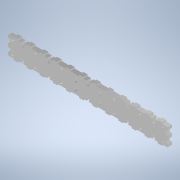
# Autodesk Inventor part: BackWallFrame
Saved by Autodesk Inventor 2021 (Build 250183000, 183)
## iProperties
Created: 2021-03-05
Part Number: BackWallFrame
Material: Aluminum 6061
Document SubType Name: Modeling
Designer: M3rob
Mass: 6286.27 g
Surface Area: 2801.63 cm^2
Volume: 2328.25 cm^3
Density: 2.7 g/cm^3
Appearance: Aluminum - Flat
Author: M3rob
Autodesk Inventor part; units mm, degrees
ref_plane "YZ Plane" through (0, 0, 0) normal (1, 0, 0) x (0, 1, 0)
ref_plane "XZ Plane" through (0, 0, 0) normal (0, 1, 0) x (-1, 0, 0)
ref_plane "XY Plane" through (0, 0, 0) normal (0, 0, 1) x (1, 0, 0)
sketch "Sketch1" plane through (0, 0, 0) normal (0, 0, 1) x (1, 0, 0)
  line L0 (-463.55, 50.8) -> (-431.8, 50.8)
  line L1 (463.55, 50.8) -> (463.55, 34.8615)
  line L2 (463.55, -50.8) -> (-463.55, -50.8)
  line L3 (-463.55, -50.8) -> (-463.55, -34.8615)
  line L4 (-463.55, 34.8615) -> (-450.85, 34.8615)
  line L5 (-450.85, 34.8615) -> (-450.85, 9.4615)
  line L6 (-450.85, 9.4615) -> (-463.55, 9.4615)
  line L7 (-463.55, -9.4615) -> (-450.85, -9.4615)
  line L8 (-450.85, -9.4615) -> (-450.85, -34.8615)
  line L9 (-450.85, -34.8615) -> (-463.55, -34.8615)
  line L10 (-463.55, 0) -> (0, 0) construction
  line L11 (0, 0) -> (0, 50.8) construction
  line L12 (-463.55, 34.8615) -> (-463.55, 50.8)
  line L13 (-463.55, 9.4615) -> (-463.55, 34.8615) construction
  line L14 (-463.55, -9.4615) -> (-463.55, 9.4615)
  line L15 (-463.55, -34.8615) -> (-463.55, -9.4615) construction
  line L16 (463.55, 34.8615) -> (450.85, 34.8615)
  line L17 (450.85, 34.8615) -> (450.85, 9.4615)
  line L18 (450.85, 9.4615) -> (463.55, 9.4615)
  line L19 (463.55, -9.4615) -> (450.85, -9.4615)
  line L20 (450.85, -9.4615) -> (450.85, -34.8615)
  line L21 (450.85, -34.8615) -> (463.55, -34.8615)
  line L22 (463.55, 9.4615) -> (463.55, -9.4615)
  line L23 (463.55, 34.8615) -> (463.55, 9.4615) construction
  line L24 (463.55, -9.4615) -> (463.55, -34.8615) construction
  line L25 (463.55, -34.8615) -> (463.55, -50.8)
  line L26 (-76.2, 34.8615) -> (-63.5, 34.8615)
  line L27 (-63.5, 34.8615) -> (-63.5, 9.4615)
  line L28 (-63.5, 9.4615) -> (-76.2, 9.4615)
  line L29 (-76.2, 9.4615) -> (-76.2, 34.8615)
  line L30 (-76.2, -9.4615) -> (-63.5, -9.4615)
  line L31 (-63.5, -9.4615) -> (-63.5, -34.8615)
  line L32 (-63.5, -34.8615) -> (-76.2, -34.8615)
  line L33 (-76.2, -34.8615) -> (-76.2, -9.4615)
  line L34 (76.2, -9.4615) -> (63.5, -9.4615)
  line L35 (63.5, -9.4615) -> (63.5, -34.8615)
  line L36 (63.5, -34.8615) -> (76.2, -34.8615)
  line L37 (76.2, -34.8615) -> (76.2, -9.4615)
  line L38 (76.2, 34.8615) -> (63.5, 34.8615)
  line L39 (63.5, 34.8615) -> (63.5, 9.4615)
  line L40 (63.5, 9.4615) -> (76.2, 9.4615)
  line L41 (76.2, 9.4615) -> (76.2, 34.8615)
  line L42 (-431.8, 50.8) -> (-431.8, 58.7375)
  line L43 (-431.8, 58.7375) -> (-406.4, 58.7375)
  line L44 (-406.4, 58.7375) -> (-406.4, 50.8)
  line L45 (-355.6, 50.8) -> (-355.6, 58.7375)
  line L46 (-355.6, 58.7375) -> (-330.2, 58.7375)
  line L47 (-330.2, 58.7375) -> (-330.2, 50.8)
  line L48 (-279.4, 50.8) -> (-279.4, 58.7375)
  line L49 (-279.4, 58.7375) -> (-254, 58.7375)
  line L50 (-254, 58.7375) -> (-254, 50.8)
  line L51 (-203.2, 50.8) -> (-203.2, 58.7375)
  line L52 (-203.2, 58.7375) -> (-177.8, 58.7375)
  line L53 (-177.8, 58.7375) -> (-177.8, 50.8)
  line L54 (-431.8, 50.8) -> (-406.4, 50.8) construction
  line L55 (-406.4, 50.8) -> (-387.7437, 50.8)
  line L56 (-355.6, 50.8) -> (-330.2, 50.8) construction
  line L57 (-330.2, 50.8) -> (-279.4, 50.8)
  line L58 (-254, 50.8) -> (-203.2, 50.8)
  line L59 (-279.4, 50.8) -> (-254, 50.8) construction
  line L60 (-177.8, 50.8) -> (463.55, 50.8)
  line L61 (-203.2, 50.8) -> (-177.8, 50.8) construction
  line L62 (-127, 58.7375) -> (-101.6, 58.7375)
  line L63 (-101.6, 58.7375) -> (-101.6, 50.8)
  line L64 (-101.6, 50.8) -> (-127, 50.8)
  line L65 (-127, 50.8) -> (-127, 50.8)
  line L66 (-127, 50.8) -> (-127, 58.7375)
  line L67 (-50.8, 50.8) -> (-50.8, 58.7375)
  line L68 (-50.8, 50.8) -> (-50.8, 50.8)
  line L69 (-25.4, 50.8) -> (-50.8, 50.8)
  line L70 (-25.4, 58.7375) -> (-25.4, 50.8)
  line L71 (-50.8, 58.7375) -> (-25.4, 58.7375)
  line L72 (25.4, 50.8) -> (25.4, 58.7375)
  line L73 (25.4, 50.8) -> (25.4, 50.8)
  line L74 (50.8, 50.8) -> (25.4, 50.8)
  line L75 (50.8, 58.7375) -> (50.8, 50.8)
  line L76 (25.4, 58.7375) -> (50.8, 58.7375)
  line L77 (101.6, 50.8) -> (101.6, 58.7375)
  line L78 (101.6, 50.8) -> (101.6, 50.8)
  line L79 (127, 50.8) -> (101.6, 50.8)
  line L80 (127, 58.7375) -> (127, 50.8)
  line L81 (101.6, 58.7375) -> (127, 58.7375)
  line L82 (177.8, 50.8) -> (177.8, 58.7375)
  line L83 (177.8, 50.8) -> (177.8, 50.8)
  line L84 (203.2, 50.8) -> (177.8, 50.8)
  line L85 (203.2, 58.7375) -> (203.2, 50.8)
  line L86 (177.8, 58.7375) -> (203.2, 58.7375)
  line L87 (254, 50.8) -> (254, 58.7375)
  line L88 (254, 50.8) -> (254, 50.8)
  line L89 (279.4, 50.8) -> (254, 50.8)
  line L90 (279.4, 58.7375) -> (279.4, 50.8)
  line L91 (254, 58.7375) -> (279.4, 58.7375)
  line L92 (330.2, 50.8) -> (330.2, 58.7375)
  line L93 (330.2, 50.8) -> (330.2, 50.8)
  line L94 (355.6, 50.8) -> (330.2, 50.8)
  line L95 (355.6, 58.7375) -> (355.6, 50.8)
  line L96 (330.2, 58.7375) -> (355.6, 58.7375)
  line L97 (406.4, 50.8) -> (406.4, 58.7375)
  line L98 (406.4, 50.8) -> (406.4, 50.8)
  line L99 (431.8, 50.8) -> (406.4, 50.8)
  line L100 (431.8, 58.7375) -> (431.8, 50.8)
  line L101 (406.4, 58.7375) -> (431.8, 58.7375)
  line L102 (431.8, 58.7375) -> (463.55, 50.8) construction
  line L103 (-431.8, 58.7375) -> (-463.55, 50.8) construction
  line L104 (-431.8, -50.8) -> (-431.8, -58.7375)
  line L105 (-431.8, -58.7375) -> (-406.4, -58.7375)
  line L106 (-406.4, -58.7375) -> (-406.4, -50.8)
  line L107 (-355.6, -50.8) -> (-355.6, -58.7375)
  line L108 (-355.6, -58.7375) -> (-330.2, -58.7375)
  line L109 (-330.2, -58.7375) -> (-330.2, -50.8)
  line L110 (-279.4, -50.8) -> (-279.4, -58.7375)
  line L111 (-279.4, -58.7375) -> (-254, -58.7375)
  line L112 (-254, -58.7375) -> (-254, -50.8)
  line L113 (-203.2, -50.8) -> (-203.2, -58.7375)
  line L114 (-203.2, -58.7375) -> (-177.8, -58.7375)
  line L115 (-177.8, -58.7375) -> (-177.8, -50.8)
  line L116 (-431.8, -50.8) -> (-406.4, -50.8) construction
  line L117 (-355.6, -50.8) -> (-330.2, -50.8) construction
  line L118 (-279.4, -50.8) -> (-254, -50.8) construction
  line L119 (-203.2, -50.8) -> (-177.8, -50.8) construction
  line L120 (-127, -58.7375) -> (-101.6, -58.7375)
  line L121 (-101.6, -58.7375) -> (-101.6, -50.8)
  line L122 (-101.6, -50.8) -> (-127, -50.8)
  line L123 (-127, -50.8) -> (-127, -58.7375)
  line L124 (-50.8, -50.8) -> (-50.8, -58.7375)
  line L125 (-25.4, -50.8) -> (-50.8, -50.8)
  line L126 (-25.4, -58.7375) -> (-25.4, -50.8)
  line L127 (-50.8, -58.7375) -> (-25.4, -58.7375)
  line L128 (25.4, -50.8) -> (25.4, -58.7375)
  line L129 (50.8, -50.8) -> (25.4, -50.8)
  line L130 (50.8, -58.7375) -> (50.8, -50.8)
  line L131 (25.4, -58.7375) -> (50.8, -58.7375)
  line L132 (101.6, -50.8) -> (101.6, -58.7375)
  line L133 (127, -50.8) -> (101.6, -50.8)
  line L134 (127, -58.7375) -> (127, -50.8)
  line L135 (101.6, -58.7375) -> (127, -58.7375)
  line L136 (177.8, -50.8) -> (177.8, -58.7375)
  line L137 (203.2, -50.8) -> (177.8, -50.8)
  line L138 (203.2, -58.7375) -> (203.2, -50.8)
  line L139 (177.8, -58.7375) -> (203.2, -58.7375)
  line L140 (254, -50.8) -> (254, -58.7375)
  line L141 (279.4, -50.8) -> (254, -50.8)
  line L142 (279.4, -58.7375) -> (279.4, -50.8)
  line L143 (254, -58.7375) -> (279.4, -58.7375)
  line L144 (330.2, -50.8) -> (330.2, -58.7375)
  line L145 (355.6, -50.8) -> (330.2, -50.8)
  line L146 (355.6, -58.7375) -> (355.6, -50.8)
  line L147 (330.2, -58.7375) -> (355.6, -58.7375)
  line L148 (406.4, -50.8) -> (406.4, -58.7375)
  line L149 (431.8, -50.8) -> (406.4, -50.8)
  line L150 (431.8, -58.7375) -> (431.8, -50.8)
  line L151 (406.4, -58.7375) -> (431.8, -58.7375)
  line L152 (-387.7437, 50.8) -> (-387.7437, 41.275)
  line L153 (-387.7437, 41.275) -> (-390.525, 41.275)
  line L154 (-390.525, 41.275) -> (-390.525, 30.1625)
  line L155 (-390.525, 30.1625) -> (-387.7437, 30.1625)
  line L156 (-387.7437, 30.1625) -> (-387.7437, 26.9875)
  line L157 (-387.7437, 26.9875) -> (-374.2563, 26.9875)
  line L158 (-374.2563, 26.9875) -> (-374.2563, 30.1625)
  line L159 (-374.2563, 30.1625) -> (-371.475, 30.1625)
  line L160 (-371.475, 30.1625) -> (-371.475, 41.275)
  line L161 (-371.475, 41.275) -> (-374.2563, 41.275)
  line L162 (-381, 50.8) -> (-381, 26.9875) construction
  line L163 (-374.2563, 41.275) -> (-374.2563, 50.8)
  line L164 (-387.7437, 50.8) -> (-374.2563, 50.8)
  line L165 (-374.2563, 50.8) -> (-355.6, 50.8)
  line L166 (-387.7437, -50.8) -> (-387.7437, -41.275)
  line L167 (-387.7437, -41.275) -> (-390.525, -41.275)
  line L168 (-390.525, -41.275) -> (-390.525, -30.1625)
  line L169 (-390.525, -30.1625) -> (-387.7437, -30.1625)
  line L170 (-387.7437, -30.1625) -> (-387.7437, -26.9875)
  line L171 (-387.7437, -26.9875) -> (-374.2563, -26.9875)
  line L172 (-374.2563, -26.9875) -> (-374.2563, -30.1625)
  line L173 (-374.2563, -30.1625) -> (-371.475, -30.1625)
  line L174 (-371.475, -30.1625) -> (-371.475, -41.275)
  line L175 (-371.475, -41.275) -> (-374.2563, -41.275)
  line L176 (-381, -50.8) -> (-381, -26.9875) construction
  line L177 (-374.2563, -41.275) -> (-374.2563, -50.8)
  line L178 (-387.7437, -50.8) -> (-374.2563, -50.8)
  line L179 (-314.325, 41.275) -> (-314.325, 30.1625)
  line L180 (-314.325, 30.1625) -> (-311.5437, 30.1625)
  line L181 (-311.5437, 30.1625) -> (-311.5437, 26.9875)
  line L182 (-304.8, 50.8) -> (-304.8, 26.9875) construction
  line L183 (-311.5437, 50.8) -> (-298.0563, 50.8)
  line L184 (-298.0563, 41.275) -> (-298.0563, 50.8)
  line L185 (-311.5437, 26.9875) -> (-298.0563, 26.9875)
  line L186 (-298.0563, 26.9875) -> (-298.0563, 30.1625)
  line L187 (-298.0563, 30.1625) -> (-295.275, 30.1625)
  line L188 (-295.275, 30.1625) -> (-295.275, 41.275)
  line L189 (-295.275, 41.275) -> (-298.0563, 41.275)
  line L190 (-311.5437, 50.8) -> (-311.5437, 41.275)
  line L191 (-311.5437, 41.275) -> (-314.325, 41.275)
  line L192 (-311.5437, -41.275) -> (-314.325, -41.275)
  line L193 (-311.5437, -50.8) -> (-311.5437, -41.275)
  line L194 (-314.325, -41.275) -> (-314.325, -30.1625)
  line L195 (-314.325, -30.1625) -> (-311.5437, -30.1625)
  line L196 (-311.5437, -30.1625) -> (-311.5437, -26.9875)
  line L197 (-311.5437, -50.8) -> (-298.0563, -50.8)
  line L198 (-304.8, -50.8) -> (-304.8, -26.9875) construction
  line L199 (-298.0563, -41.275) -> (-298.0563, -50.8)
  line L200 (-295.275, -41.275) -> (-298.0563, -41.275)
  line L201 (-311.5437, -26.9875) -> (-298.0563, -26.9875)
  line L202 (-295.275, -30.1625) -> (-295.275, -41.275)
  line L203 (-298.0563, -30.1625) -> (-295.275, -30.1625)
  line L204 (-298.0563, -26.9875) -> (-298.0563, -30.1625)
  line L205 (-238.125, 41.275) -> (-238.125, 30.1625)
  line L206 (-238.125, 30.1625) -> (-235.3437, 30.1625)
  line L207 (-235.3437, 30.1625) -> (-235.3437, 26.9875)
  line L208 (-228.6, 50.8) -> (-228.6, 26.9875) construction
  line L209 (-235.3437, 50.8) -> (-221.8563, 50.8)
  line L210 (-221.8563, 41.275) -> (-221.8563, 50.8)
  line L211 (-235.3437, 26.9875) -> (-221.8563, 26.9875)
  line L212 (-221.8563, 26.9875) -> (-221.8563, 30.1625)
  line L213 (-221.8563, 30.1625) -> (-219.075, 30.1625)
  line L214 (-219.075, 30.1625) -> (-219.075, 41.275)
  line L215 (-219.075, 41.275) -> (-221.8563, 41.275)
  line L216 (-235.3437, 50.8) -> (-235.3437, 41.275)
  line L217 (-235.3437, 41.275) -> (-238.125, 41.275)
  line L218 (-235.3437, -41.275) -> (-238.125, -41.275)
  line L219 (-235.3437, -50.8) -> (-235.3437, -41.275)
  line L220 (-238.125, -41.275) -> (-238.125, -30.1625)
  line L221 (-238.125, -30.1625) -> (-235.3437, -30.1625)
  line L222 (-235.3437, -30.1625) -> (-235.3437, -26.9875)
  line L223 (-235.3437, -50.8) -> (-221.8563, -50.8)
  line L224 (-228.6, -50.8) -> (-228.6, -26.9875) construction
  line L225 (-221.8563, -41.275) -> (-221.8563, -50.8)
  line L226 (-219.075, -41.275) -> (-221.8563, -41.275)
  line L227 (-235.3437, -26.9875) -> (-221.8563, -26.9875)
  line L228 (-219.075, -30.1625) -> (-219.075, -41.275)
  line L229 (-221.8563, -30.1625) -> (-219.075, -30.1625)
  line L230 (-221.8563, -26.9875) -> (-221.8563, -30.1625)
  line L231 (-161.925, 41.275) -> (-161.925, 30.1625)
  line L232 (-161.925, 30.1625) -> (-159.1437, 30.1625)
  line L233 (-159.1437, 30.1625) -> (-159.1437, 26.9875)
  line L234 (-152.4, 50.8) -> (-152.4, 26.9875) construction
  line L235 (-159.1437, 50.8) -> (-145.6563, 50.8)
  line L236 (-145.6563, 41.275) -> (-145.6563, 50.8)
  line L237 (-159.1437, 26.9875) -> (-145.6563, 26.9875)
  line L238 (-145.6563, 26.9875) -> (-145.6563, 30.1625)
  line L239 (-145.6563, 30.1625) -> (-142.875, 30.1625)
  line L240 (-142.875, 30.1625) -> (-142.875, 41.275)
  line L241 (-142.875, 41.275) -> (-145.6563, 41.275)
  line L242 (-159.1437, 50.8) -> (-159.1437, 41.275)
  line L243 (-159.1437, 41.275) -> (-161.925, 41.275)
  line L244 (-159.1437, -41.275) -> (-161.925, -41.275)
  line L245 (-159.1437, -50.8) -> (-159.1437, -41.275)
  line L246 (-161.925, -41.275) -> (-161.925, -30.1625)
  line L247 (-161.925, -30.1625) -> (-159.1437, -30.1625)
  line L248 (-159.1437, -30.1625) -> (-159.1437, -26.9875)
  line L249 (-159.1437, -50.8) -> (-145.6563, -50.8)
  line L250 (-152.4, -50.8) -> (-152.4, -26.9875) construction
  line L251 (-145.6563, -41.275) -> (-145.6563, -50.8)
  line L252 (-142.875, -41.275) -> (-145.6563, -41.275)
  line L253 (-159.1437, -26.9875) -> (-145.6563, -26.9875)
  line L254 (-142.875, -30.1625) -> (-142.875, -41.275)
  line L255 (-145.6563, -30.1625) -> (-142.875, -30.1625)
  line L256 (-145.6563, -26.9875) -> (-145.6563, -30.1625)
  line L257 (-85.725, 41.275) -> (-85.725, 30.1625)
  line L258 (-85.725, 30.1625) -> (-82.9437, 30.1625)
  line L259 (-82.9437, 30.1625) -> (-82.9437, 26.9875)
  line L260 (-76.2, 50.8) -> (-76.2, 26.9875) construction
  line L261 (-82.9437, 50.8) -> (-69.4563, 50.8)
  line L262 (-69.4563, 41.275) -> (-69.4563, 50.8)
  line L263 (-82.9437, 26.9875) -> (-69.4563, 26.9875)
  line L264 (-69.4563, 26.9875) -> (-69.4563, 30.1625)
  line L265 (-69.4563, 30.1625) -> (-66.675, 30.1625)
  line L266 (-66.675, 30.1625) -> (-66.675, 41.275)
  line L267 (-66.675, 41.275) -> (-69.4563, 41.275)
  line L268 (-82.9437, 50.8) -> (-82.9437, 41.275)
  line L269 (-82.9437, 41.275) -> (-85.725, 41.275)
  line L270 (-82.9437, -41.275) -> (-85.725, -41.275)
  line L271 (-82.9437, -50.8) -> (-82.9437, -41.275)
  line L272 (-85.725, -41.275) -> (-85.725, -30.1625)
  line L273 (-85.725, -30.1625) -> (-82.9437, -30.1625)
  line L274 (-82.9437, -30.1625) -> (-82.9437, -26.9875)
  line L275 (-82.9437, -50.8) -> (-69.4563, -50.8)
  line L276 (-76.2, -50.8) -> (-76.2, -26.9875) construction
  line L277 (-69.4563, -41.275) -> (-69.4563, -50.8)
  line L278 (-66.675, -41.275) -> (-69.4563, -41.275)
  line L279 (-82.9437, -26.9875) -> (-69.4563, -26.9875)
  line L280 (-66.675, -30.1625) -> (-66.675, -41.275)
  line L281 (-69.4563, -30.1625) -> (-66.675, -30.1625)
  line L282 (-69.4563, -26.9875) -> (-69.4563, -30.1625)
  line L283 (-9.525, 41.275) -> (-9.525, 30.1625)
  line L284 (-9.525, 30.1625) -> (-6.7437, 30.1625)
  line L285 (-6.7437, 30.1625) -> (-6.7437, 26.9875)
  line L286 (0, 50.8) -> (0, 26.9875) construction
  line L287 (-6.7437, 50.8) -> (6.7437, 50.8)
  line L288 (6.7437, 41.275) -> (6.7437, 50.8)
  line L289 (-6.7437, 26.9875) -> (6.7437, 26.9875)
  line L290 (6.7437, 26.9875) -> (6.7437, 30.1625)
  line L291 (6.7437, 30.1625) -> (9.525, 30.1625)
  line L292 (9.525, 30.1625) -> (9.525, 41.275)
  line L293 (9.525, 41.275) -> (6.7437, 41.275)
  line L294 (-6.7437, 50.8) -> (-6.7437, 41.275)
  line L295 (-6.7437, 41.275) -> (-9.525, 41.275)
  line L296 (-6.7437, -41.275) -> (-9.525, -41.275)
  line L297 (-6.7437, -50.8) -> (-6.7437, -41.275)
  line L298 (-9.525, -41.275) -> (-9.525, -30.1625)
  line L299 (-9.525, -30.1625) -> (-6.7437, -30.1625)
  line L300 (-6.7437, -30.1625) -> (-6.7437, -26.9875)
  line L301 (-6.7437, -50.8) -> (6.7437, -50.8)
  line L302 (0, -50.8) -> (0, -26.9875) construction
  line L303 (6.7437, -41.275) -> (6.7437, -50.8)
  line L304 (9.525, -41.275) -> (6.7437, -41.275)
  line L305 (-6.7437, -26.9875) -> (6.7437, -26.9875)
  line L306 (9.525, -30.1625) -> (9.525, -41.275)
  line L307 (6.7437, -30.1625) -> (9.525, -30.1625)
  line L308 (6.7437, -26.9875) -> (6.7437, -30.1625)
  line L309 (66.675, 41.275) -> (66.675, 30.1625)
  line L310 (66.675, 30.1625) -> (69.4563, 30.1625)
  line L311 (69.4563, 30.1625) -> (69.4563, 26.9875)
  line L312 (76.2, 50.8) -> (76.2, 26.9875) construction
  line L313 (69.4563, 50.8) -> (82.9437, 50.8)
  line L314 (82.9437, 41.275) -> (82.9437, 50.8)
  line L315 (69.4563, 26.9875) -> (82.9437, 26.9875)
  line L316 (82.9437, 26.9875) -> (82.9437, 30.1625)
  line L317 (82.9437, 30.1625) -> (85.725, 30.1625)
  line L318 (85.725, 30.1625) -> (85.725, 41.275)
  line L319 (85.725, 41.275) -> (82.9437, 41.275)
  line L320 (69.4563, 50.8) -> (69.4563, 41.275)
  line L321 (69.4563, 41.275) -> (66.675, 41.275)
  line L322 (69.4563, -41.275) -> (66.675, -41.275)
  line L323 (69.4563, -50.8) -> (69.4563, -41.275)
  line L324 (66.675, -41.275) -> (66.675, -30.1625)
  line L325 (66.675, -30.1625) -> (69.4563, -30.1625)
  line L326 (69.4563, -30.1625) -> (69.4563, -26.9875)
  line L327 (69.4563, -50.8) -> (82.9437, -50.8)
  line L328 (76.2, -50.8) -> (76.2, -26.9875) construction
  line L329 (82.9437, -41.275) -> (82.9437, -50.8)
  line L330 (85.725, -41.275) -> (82.9437, -41.275)
  line L331 (69.4563, -26.9875) -> (82.9437, -26.9875)
  line L332 (85.725, -30.1625) -> (85.725, -41.275)
  line L333 (82.9437, -30.1625) -> (85.725, -30.1625)
  line L334 (82.9437, -26.9875) -> (82.9437, -30.1625)
  line L335 (142.875, 41.275) -> (142.875, 30.1625)
  line L336 (142.875, 30.1625) -> (145.6563, 30.1625)
  line L337 (145.6563, 30.1625) -> (145.6563, 26.9875)
  line L338 (152.4, 50.8) -> (152.4, 26.9875) construction
  line L339 (145.6563, 50.8) -> (159.1437, 50.8)
  line L340 (159.1437, 41.275) -> (159.1437, 50.8)
  line L341 (145.6563, 26.9875) -> (159.1437, 26.9875)
  line L342 (159.1437, 26.9875) -> (159.1437, 30.1625)
  line L343 (159.1437, 30.1625) -> (161.925, 30.1625)
  line L344 (161.925, 30.1625) -> (161.925, 41.275)
  line L345 (161.925, 41.275) -> (159.1437, 41.275)
  line L346 (145.6563, 50.8) -> (145.6563, 41.275)
  line L347 (145.6563, 41.275) -> (142.875, 41.275)
  line L348 (145.6563, -41.275) -> (142.875, -41.275)
  line L349 (145.6563, -50.8) -> (145.6563, -41.275)
  line L350 (142.875, -41.275) -> (142.875, -30.1625)
  line L351 (142.875, -30.1625) -> (145.6563, -30.1625)
  line L352 (145.6563, -30.1625) -> (145.6563, -26.9875)
  line L353 (145.6563, -50.8) -> (159.1437, -50.8)
  line L354 (152.4, -50.8) -> (152.4, -26.9875) construction
  line L355 (159.1437, -41.275) -> (159.1437, -50.8)
  line L356 (161.925, -41.275) -> (159.1437, -41.275)
  line L357 (145.6563, -26.9875) -> (159.1437, -26.9875)
  line L358 (161.925, -30.1625) -> (161.925, -41.275)
  line L359 (159.1437, -30.1625) -> (161.925, -30.1625)
  line L360 (159.1437, -26.9875) -> (159.1437, -30.1625)
  line L361 (219.075, 41.275) -> (219.075, 30.1625)
  line L362 (219.075, 30.1625) -> (221.8563, 30.1625)
  line L363 (221.8563, 30.1625) -> (221.8563, 26.9875)
  line L364 (228.6, 50.8) -> (228.6, 26.9875) construction
  line L365 (221.8563, 50.8) -> (235.3437, 50.8)
  line L366 (235.3437, 41.275) -> (235.3437, 50.8)
  line L367 (221.8563, 26.9875) -> (235.3437, 26.9875)
  line L368 (235.3437, 26.9875) -> (235.3437, 30.1625)
  line L369 (235.3437, 30.1625) -> (238.125, 30.1625)
  line L370 (238.125, 30.1625) -> (238.125, 41.275)
  line L371 (238.125, 41.275) -> (235.3437, 41.275)
  line L372 (221.8563, 50.8) -> (221.8563, 41.275)
  line L373 (221.8563, 41.275) -> (219.075, 41.275)
  line L374 (221.8563, -41.275) -> (219.075, -41.275)
  line L375 (221.8563, -50.8) -> (221.8563, -41.275)
  line L376 (219.075, -41.275) -> (219.075, -30.1625)
  line L377 (219.075, -30.1625) -> (221.8563, -30.1625)
  line L378 (221.8563, -30.1625) -> (221.8563, -26.9875)
  line L379 (221.8563, -50.8) -> (235.3437, -50.8)
  line L380 (228.6, -50.8) -> (228.6, -26.9875) construction
  line L381 (235.3437, -41.275) -> (235.3437, -50.8)
  line L382 (238.125, -41.275) -> (235.3437, -41.275)
  line L383 (221.8563, -26.9875) -> (235.3437, -26.9875)
  line L384 (238.125, -30.1625) -> (238.125, -41.275)
  line L385 (235.3437, -30.1625) -> (238.125, -30.1625)
  line L386 (235.3437, -26.9875) -> (235.3437, -30.1625)
  line L387 (295.275, 41.275) -> (295.275, 30.1625)
  line L388 (295.275, 30.1625) -> (298.0563, 30.1625)
  line L389 (298.0563, 30.1625) -> (298.0563, 26.9875)
  line L390 (304.8, 50.8) -> (304.8, 26.9875) construction
  line L391 (298.0563, 50.8) -> (311.5437, 50.8)
  line L392 (311.5437, 41.275) -> (311.5437, 50.8)
  line L393 (298.0563, 26.9875) -> (311.5437, 26.9875)
  line L394 (311.5437, 26.9875) -> (311.5437, 30.1625)
  line L395 (311.5437, 30.1625) -> (314.325, 30.1625)
  line L396 (314.325, 30.1625) -> (314.325, 41.275)
  line L397 (314.325, 41.275) -> (311.5437, 41.275)
  line L398 (298.0563, 50.8) -> (298.0563, 41.275)
  line L399 (298.0563, 41.275) -> (295.275, 41.275)
  line L400 (298.0563, -41.275) -> (295.275, -41.275)
  line L401 (298.0563, -50.8) -> (298.0563, -41.275)
  line L402 (295.275, -41.275) -> (295.275, -30.1625)
  line L403 (295.275, -30.1625) -> (298.0563, -30.1625)
  line L404 (298.0563, -30.1625) -> (298.0563, -26.9875)
  line L405 (298.0563, -50.8) -> (311.5437, -50.8)
  line L406 (304.8, -50.8) -> (304.8, -26.9875) construction
  line L407 (311.5437, -41.275) -> (311.5437, -50.8)
  line L408 (314.325, -41.275) -> (311.5437, -41.275)
  line L409 (298.0563, -26.9875) -> (311.5437, -26.9875)
  line L410 (314.325, -30.1625) -> (314.325, -41.275)
  line L411 (311.5437, -30.1625) -> (314.325, -30.1625)
  line L412 (311.5437, -26.9875) -> (311.5437, -30.1625)
  line L413 (371.475, 41.275) -> (371.475, 30.1625)
  line L414 (371.475, 30.1625) -> (374.2563, 30.1625)
  line L415 (374.2563, 30.1625) -> (374.2563, 26.9875)
  line L416 (381, 50.8) -> (381, 26.9875) construction
  line L417 (374.2563, 50.8) -> (387.7437, 50.8)
  line L418 (387.7437, 41.275) -> (387.7437, 50.8)
  line L419 (374.2563, 26.9875) -> (387.7437, 26.9875)
  line L420 (387.7437, 26.9875) -> (387.7437, 30.1625)
  line L421 (387.7437, 30.1625) -> (390.525, 30.1625)
  line L422 (390.525, 30.1625) -> (390.525, 41.275)
  line L423 (390.525, 41.275) -> (387.7437, 41.275)
  line L424 (374.2563, 50.8) -> (374.2563, 41.275)
  line L425 (374.2563, 41.275) -> (371.475, 41.275)
  line L426 (374.2563, -41.275) -> (371.475, -41.275)
  line L427 (374.2563, -50.8) -> (374.2563, -41.275)
  line L428 (371.475, -41.275) -> (371.475, -30.1625)
  line L429 (371.475, -30.1625) -> (374.2563, -30.1625)
  line L430 (374.2563, -30.1625) -> (374.2563, -26.9875)
  line L431 (374.2563, -50.8) -> (387.7437, -50.8)
  line L432 (381, -50.8) -> (381, -26.9875) construction
  line L433 (387.7437, -41.275) -> (387.7437, -50.8)
  line L434 (390.525, -41.275) -> (387.7437, -41.275)
  line L435 (374.2563, -26.9875) -> (387.7437, -26.9875)
  line L436 (390.525, -30.1625) -> (390.525, -41.275)
  line L437 (387.7437, -30.1625) -> (390.525, -30.1625)
  line L438 (387.7437, -26.9875) -> (387.7437, -30.1625)
  point P0 (463.55, 0)
  point P1 (0, -50.8)
  point P2 (-66.675, 34.8615)
  point P3 (-76.2, 26.9875)
  dimension "d0" = 927.1
  dimension "d1" = 101.6
  dimension "d2" = 12.7
  dimension "d3" = 25.4
  dimension "d4" = 18.923
  dimension "d7" = 127
  dimension "d8" = 12.7
  dimension "d9" = 25.4
  dimension "d10" = 50.8
  dimension "d11" = 7.9375
  dimension "d12" = 50.8
  dimension "d15" = 76.2
  dimension "d20" = 9.525
  dimension "d21" = 11.1125
  dimension "d22" = 3.175
  dimension "d23" = 19.05
  dimension "d24" = 13.4874
  dimension "d25" = 50.8
  dimension "d28" = 76.2
  constraints: 872 end point, 204 point on line, 107 perpendicular, 70 symmetric about line, 62 parallel, 41 horizontal alignment, 27 horizontal, 19 equal length, 18 vertical, 14 collinear, 5 vertical alignment, 1 midpoint, 564 other
  measures "d0" distance of L12.end L1.start
  measures "d1" distance of L1.start L25.end
  measures "d2" distance of L4.start L4.end
  measures "d3" distance of L4.end L5.end
  measures "d4" distance between parallel lines of L7 L6
  measures "d7" diameter of L39 L11
  measures "d8" distance of L38.start L38.end
  measures "d9" distance of L42.end L43.end
  measures "d10" distance of L45.end L43.end
  measures "d11" distance of L42.start L42.end
  measures "d12" distance of L52.end L62.start
  measures "d15" distance of L65.end L67.start
  measures "d20" distance of L161.end L163.end
  measures "d21" distance of L159.end L160.end
  measures "d22" distance of L157.end L158.end
  measures "d23" distance between parallel lines of L154 L160
  measures "d24" distance between parallel lines of L163 L152
  measures "d25" distance of L48.end L46.end
  measures "d28" distance of L154.end L179.end
extrude "Extrusion1" add sketch "Sketch1" against normal blind 25.4 contours L0 L42 L43 L44 L55 L152 L153 L154 L155 L156 L157 L158 L159 L160 L161 L163 L165 L45 L46 L47 L57 L190 L191 L179 L180 L181 L185 L186 L187 L188 L189 L184 L48 L49 L50 L58 L216 L217 L205 L206 L207 L211 L212 L213 L214 L215 L210 L51 L52 L53 L60 L242 L243 L231 L232 L233 L237 L238 L239 L240 L241 L236 L268 L269 L257 L258 L259 L263 L29 L28 L27 L26 L266 L267 L262 L294 L295 L283 L284 L285 L289 L290 L291 L292 L293 L288 L320 L321 L309 L38 L39 L40 L41 L315 L316 L317 L318 L319 L314 L346 L347 L335 L336 L337 L341 L342 L343 L344 L345 L340 L372 L373 L361 L362 L363 L367 L368 L369 L370 L371 L366 L398 L399 L387 L388 L389 L393 L394 L395 L396 L397 L392 L424 L425 L413 L414 L415 L419 L420 L421 L422 L423 L418 L1 L16 L17 L18 L22 L19 L20 L21 L25 L2 L433 L434 L436 L437 L438 L435 L430 L429 L428 L426 L427 L407 L408 L410 L411 L412 L409 L404 L403 L402 L400 L401 L381 L382 L384 L385 L386 L383 L378 L377 L376 L374 L375 L355 L356 L358 L359 L360 L357 L352 L351 L350 L348 L349 L329 L330 L332 L333 L334 L331 L37 L34 L35 L36 L324 L322 L323 L303 L304 L306 L307 L308 L305 L300 L299 L298 L296 L297 L277 L278 L280 L32 L31 L30 L33 L279 L274 L273 L272 L270 L271 L251 L252 L254 L255 L256 L253 L248 L247 L246 L244 L245 L225 L226 L228 L229 L230 L227 L222 L221 L220 L218 L219 L199 L200 L202 L203 L204 L201 L196 L195 L194 L192 L193 L177 L175 L174 L173 L172 L171 L170 L169 L168 L167 L166 L3 L9 L8 L7 L14 L6 L5 L4 L12 | L2 L106 L105 L104 | L57 L184 L189 L188 L187 L186 L185 L181 L180 L179 L191 L190 | L2 L109 L108 L107 | L193 L192 L194 L195 L196 L201 L204 L203 L202 L200 L199 L2 | L2 L112 L111 L110 | L2 L115 L114 L113 | L60 L236 L241 L240 L239 L238 L237 L233 L232 L231 L243 L242 | L245 L244 L246 L247 L248 L253 L256 L255 L254 L252 L251 L2 | L66 L62 L63 L60 | L2 L121 L120 L123 | L60 L262 L267 L266 L26 L29 L263 L259 L258 L257 L269 L268 | L271 L270 L272 L273 L274 L279 L33 L32 L280 L278 L277 L2 | L67 L71 L70 L60 | L2 L126 L127 L124 | L72 L76 L75 L60 | L2 L130 L131 L128 | L60 L314 L319 L318 L317 L316 L315 L41 L38 L309 L321 L320 | L323 L322 L324 L36 L37 L331 L334 L333 L332 L330 L329 L2 | L77 L81 L80 L60 | L2 L134 L135 L132 | L60 L340 L345 L344 L343 L342 L341 L337 L336 L335 L347 L346 | L349 L348 L350 L351 L352 L357 L360 L359 L358 L356 L355 L2 | L82 L86 L85 L60 | L2 L138 L139 L136 | L87 L91 L90 L60 | L2 L142 L143 L140 | L60 L392 L397 L396 L395 L394 L393 L389 L388 L387 L399 L398 | L401 L400 L402 L403 L404 L409 L412 L411 L410 L408 L407 L2 | L92 L96 L95 L60 | L2 L146 L147 L144 | L97 L101 L100 L60 | L2 L150 L151 L148
sketch "Sketch2" plane through (0, 0, 0) normal (0, 0, 1) x (1, 0, 0)
  circle A0 centre (-436.5625, 36.5125) radius 14.2875 construction
  circle A1 centre (-304.8, 36.5125) radius 14.2875 construction
  circle A2 centre (-152.4, 36.5125) radius 14.2875 construction
  circle A3 centre (152.4, 36.5125) radius 14.2875 construction
  circle A4 centre (304.8, 36.5125) radius 14.2875 construction
  circle A5 centre (436.5625, 36.5125) radius 14.2875 construction
  line L0 (-279.4, 50.8) -> (-330.2, 50.8) construction
  line L1 (-127, 50.8) -> (-177.8, 50.8) construction
  line L2 (177.8, 50.8) -> (127, 50.8) construction
  line L3 (330.2, 50.8) -> (279.4, 50.8) construction
  line L4 (-450.85, 34.8615) -> (-450.85, 9.4615) construction
  line L5 (-431.8, 50.8) -> (-463.55, 50.8) construction
  line L6 (463.55, 50.8) -> (431.8, 50.8) construction
  line L7 (450.85, 9.4615) -> (450.85, 34.8615) construction
  circle A6 centre (436.5625, 36.5125) radius 4.7625 construction
  line L8 (436.5625, 41.275) -> (436.5625, 50.8) construction
  line L9 (463.55, 9.4615) -> (463.55, -9.4615) construction
  line L10 (463.55, 0) -> (0, 0) construction
  circle A7 centre (-436.5625, -36.5125) radius 14.2875 construction
  circle A8 centre (-304.8, -36.5125) radius 14.2875 construction
  circle A9 centre (-152.4, -36.5125) radius 14.2875 construction
  circle A10 centre (152.4, -36.5125) radius 14.2875 construction
  circle A11 centre (304.8, -36.5125) radius 14.2875 construction
  circle A12 centre (436.5625, -36.5125) radius 14.2875 construction
  line L11 (-279.4, -50.8) -> (-330.2, -50.8) construction
  line L12 (-127, -50.8) -> (-177.8, -50.8) construction
  line L13 (177.8, -50.8) -> (127, -50.8) construction
  line L14 (330.2, -50.8) -> (279.4, -50.8) construction
  line L15 (-450.85, -34.8615) -> (-450.85, -9.4615) construction
  line L16 (-431.8, -50.8) -> (-463.55, -50.8) construction
  line L17 (463.55, -50.8) -> (431.8, -50.8) construction
  line L18 (450.85, -9.4615) -> (450.85, -34.8615) construction
  circle A13 centre (436.5625, -36.5125) radius 4.7625 construction
  line L19 (436.5625, -41.275) -> (436.5625, -50.8) construction
  point P0 (-304.8, 50.8)
  point P1 (-152.4, 50.8)
  point P2 (152.4, 50.8)
  point P3 (304.8, 50.8)
  point P4 (-304.8, -50.8)
  point P5 (-152.4, -50.8)
  point P6 (152.4, -50.8)
  point P7 (304.8, -50.8)
  dimension "d34" = 9.525
  dimension "d33" = 9.525
  constraints: 29 symmetric about line, 22 end point, 10 centre point, 8 vertical alignment, 6 tangent, 5 midpoint, 4 equal radius, 4 horizontal, 2 coincident, 2 point on line, 2 vertical, 14 other
  measures "d33" distance of L8.start L8.end
hole "Hole1" at (-436.5625, 36.5125, 0) at (-304.8, 36.5125, 0) at (-304.8, -36.5125, 0) at (-436.5625, -36.5125, 0) at (-152.4, 36.5125, 0) at (-152.4, -36.5125, 0) at (152.4, 36.5125, 0) at (152.4, -36.5125, 0) at (304.8, 36.5125, 0) at (304.8, -36.5125, 0) at (436.5625, -36.5125, 0) at (436.5625, 36.5125, 0) direction (0, 0, -1) diameter 10.0838 depth 35.179 tip angle 118 clearance for "Hex Head Bolt" size "3/8" standard "Ansi Unified Screw Threads"
body "Solid1"
